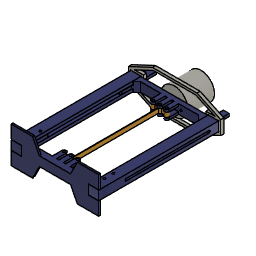
Modelo Pandeo De Columna (Autodesk Fusion 360 design; units mm, degrees)
Autodesk Fusion 360 part; units mm, degrees
note: some values were not read from the file. Set by a fixed rule: which sketch regions a step uses.
(part 1 of 2)
sketch "Boceto1" plane through (0, 0, 0) normal (0, 0, 1) x (1, 0, 0)
  circle A0 centre (0, 0) radius 2.65
  circle A1 centre (-15, 0) radius 2.65
  circle A2 centre (15, 0) radius 2.65
  circle A3 centre (0, 200) radius 2.65
  circle A4 centre (-15, 200) radius 2.65
  circle A5 centre (15, 200) radius 2.65
  line L0 (-15, 0) -> (15, 0) construction
  line L1 (-15, 200) -> (15, 200) construction
  line L2 (0, 0) -> (0, 200) construction
  line L3 (-0.5, 197.3976) -> (-0.5, 2.6024)
  line L4 (0.5, 2.6024) -> (0.5, 197.3976)
  line L5 (-12.5459, 201) -> (-2.4541, 201)
  line L6 (-12.5459, 199) -> (-2.4541, 199)
  line L7 (2.4541, 201) -> (12.5459, 201)
  line L8 (2.4541, 199) -> (12.5459, 199)
  line L9 (-12.5459, 1) -> (-2.4541, 1)
  line L10 (-12.5459, -1) -> (-2.4541, -1)
  line L11 (2.4541, 1) -> (12.5459, 1)
  line L12 (2.4541, -1) -> (12.5459, -1)
  circle A6 centre (-15, 200) radius 4.25
  circle A7 centre (0, 200) radius 4.25
  circle A8 centre (15, 200) radius 4.25
  circle A9 centre (-15, 0) radius 4.25
  circle A10 centre (0, 0) radius 4.25
  circle A11 centre (15, 0) radius 4.25
  dimension "d1" = 5.3
  dimension "d2" = 30
  dimension "d3" = 200
  dimension "Altura_Columna" = 200
  dimension "Ancho_Estructura" = 10
  dimension "Espesor_Columna" = 1
  dimension "d7" = 2
  dimension "d8" = 2
  dimension "d9" = 2
  dimension "d10" = 2
  dimension "d11" = 1
  dimension "d12" = 1.6
  dimension "d13" = 1.6
  dimension "d14" = 1.6
  dimension "d15" = 1.6
  dimension "d16" = 1.6
  dimension "d17" = 1.6
  dimension "Ancho_Columna" = 9.99
  constraint coincident A0.centre L2.start
  constraint equal A0 A1
  constraint equal A0 A2
  constraint equal A0 A3
  constraint equal A3 A4
  constraint equal A3 A5
  constraint coincident A1.centre L0.start
  constraint coincident A2.centre L0.end
  constraint coincident A4.centre L1.start
  constraint coincident A5.centre L1.end
  constraint horizontal L1
  constraint horizontal L0
  constraint coincident A0.centre L0
  constraint coincident A3.centre L1
  constraint equal L0 L1
  constraint coincident A3.centre L2.end
  constraint vertical L2
  constraint symmetric A1 A2 L2
  constraint symmetric A4 A5 L2
  constraint coincident A3 L3.start
  constraint coincident A0 L3.end
  constraint parallel L2 L3
  constraint coincident A0 L4.start
  constraint coincident A3 L4.end
  constraint parallel L2 L4
  constraint coincident A4 L5.start
  constraint coincident A3 L5.end
  constraint perpendicular L4 L5
  constraint coincident A4 L6.start
  constraint coincident A3 L6.end
  constraint parallel L5 L6
  constraint coincident A3 L7.start
  constraint coincident A5 L7.end
  constraint perpendicular L2 L7
  constraint coincident A3 L8.start
  constraint coincident A5 L8.end
  constraint perpendicular L2 L8
  constraint equal L5 L6
  constraint equal L7 L8
  constraint equal L3 L4
  constraint coincident A1 L9.start
  constraint coincident A0 L9.end
  constraint parallel L0 L9
  constraint coincident A1 L10.start
  constraint coincident A0 L10.end
  constraint parallel L0 L10
  constraint coincident A0 L11.start
  constraint coincident A2 L11.end
  constraint parallel L10 L11
  constraint coincident A0 L12.start
  constraint coincident A2 L12.end
  constraint parallel L0 L12
  constraint equal L9 L10
  constraint equal L11 L12
  measures "d1" diameter of A0
  measures "d2" distance of A1.centre A2.centre
  measures "d3" distance of A0.centre A3.centre
  measures "d7" distance of L5 L6
  measures "d8" distance of L7 L8
  measures "d9" distance of L11 L12
  measures "d10" distance of L9 L10
  measures "d11" distance of L3 L4
extrude "Extruir1" add sketch "Boceto1" along normal blind 10 contours A0 L11 L12 A10 | A0 L4 L11 A10 | A0 L10 L12 A10 | A0 L3 L4 A10 | L11 L12 A10 A11 | A0 L9 L10 A10 | A0 L3 L9 A10 | L3 L4 A7 A10 | A2 L11 L12 A11 | A2 L11 L12 A11 | L9 L10 A9 A10 | A3 L3 L4 A7 | A3 L4 L8 A7 | A1 L9 L10 A9 | A1 L9 L10 A9 | A3 L3 L6 A7 | L7 L8 A7 A8 | A3 L7 L8 A7 | A3 L5 L6 A7 | L5 L6 A6 A7 | A5 L7 L8 A8 | A5 L7 L8 A8 | A4 L5 L6 A6 | A4 L5 L6 A6 | A3 L5 L7 A7 makes body 1
ref_plane "PlanoDeObra1" through (0, 100, 10.4) normal (0, 0, 1) x (1, 0, 0)
sketch "Boceto2" plane through (0, 0, 10.4) normal (0, 0, 1) x (1, 0, 0)
  line L0 (10.8693, 1) -> (4.1307, 1)
  arc A0 (4.1307, 1) -> (0.5, 4.2205) centre (0, 0) ccw
  line L1 (0.5, 4.2205) -> (0.5, 195.7795)
  line L2 (-95, 221.5) -> (95, 221.5)
  line L3 (0, 200) -> (0, 221.5) construction
  line L4 (-95, -21.5) -> (95, -21.5)
  line L5 (0, 0) -> (0, -21.5) construction
  line L6 (-95, 221.5) -> (-95, 231.5)
  line L7 (-95, 231.5) -> (95, 231.5)
  line L8 (95, 231.5) -> (95, 221.5)
  line L9 (-95, -21.5) -> (-95, -31.5)
  line L10 (-95, -31.5) -> (95, -31.5)
  line L11 (95, -31.5) -> (95, -21.5)
  circle A1 centre (-15, 200) radius 5
  circle A2 centre (15, 200) radius 5
  circle A3 centre (0, 200) radius 5
  circle A4 centre (-15, 0) radius 5
  circle A5 centre (0, 0) radius 5
  circle A6 centre (15, 0) radius 5
  line L12 (-20, 0) -> (-10, 0) construction
  line L13 (-10, 0) -> (-10, -21.5)
  line L14 (-10, -21.5) -> (-20, -21.5)
  line L15 (-20, -21.5) -> (-20, 0)
  line L16 (-5, 0) -> (5, 0) construction
  line L17 (5, 0) -> (5, -21.5)
  line L18 (5, -21.5) -> (-5, -21.5)
  line L19 (-5, -21.5) -> (-5, 0)
  line L20 (10, 0) -> (20, 0) construction
  line L21 (20, 0) -> (20, -21.5)
  line L22 (20, -21.5) -> (10, -21.5)
  line L23 (10, -21.5) -> (10, 0)
  line L24 (-20, 200) -> (-10, 200) construction
  line L25 (-10, 200) -> (-10, 221.5)
  line L26 (-10, 221.5) -> (-20, 221.5)
  line L27 (-20, 221.5) -> (-20, 200)
  line L28 (-5, 200) -> (5, 200) construction
  line L29 (5, 200) -> (5, 221.5)
  line L30 (5, 221.5) -> (-5, 221.5)
  line L31 (-5, 221.5) -> (-5, 200)
  line L32 (10, 200) -> (20, 200) construction
  line L33 (20, 200) -> (20, 221.5)
  line L34 (20, 221.5) -> (10, 221.5)
  line L35 (10, 221.5) -> (10, 200)
  circle A7 centre (15, 200) radius 2.65
  circle A8 centre (-15, 200) radius 2.65
  circle A9 centre (0, 200) radius 2.65
  circle A10 centre (15, 0) radius 2.65
  circle A11 centre (-15, 0) radius 2.65
  circle A12 centre (0, 0) radius 2.65
  arc A13 (-10.8693, 1) -> (-10.8693, -1) centre (-15, 0) ccw
  line L36 (-10.8693, -1) -> (-4.1307, -1)
  arc A14 (-4.1307, -1) -> (4.1307, -1) centre (0, 0) ccw
  line L37 (4.1307, -1) -> (10.8693, -1)
  arc A15 (10.8693, -1) -> (10.8693, 1) centre (15, 0) ccw
  arc A16 (0.5, 195.7795) -> (4.1307, 199) centre (0, 200) ccw
  line L38 (4.1307, 199) -> (10.8693, 199)
  arc A17 (10.8693, 199) -> (10.8693, 201) centre (15, 200) ccw
  line L39 (10.8693, 201) -> (4.1307, 201)
  arc A18 (4.1307, 201) -> (-4.1307, 201) centre (0, 200) ccw
  line L40 (-4.1307, 201) -> (-10.8693, 201)
  arc A19 (-10.8693, 201) -> (-10.8693, 199) centre (-15, 200) ccw
  line L41 (-10.8693, 199) -> (-4.1307, 199)
  arc A20 (-4.1307, 199) -> (-0.5, 195.7795) centre (0, 200) ccw
  line L42 (-0.5, 195.7795) -> (-0.5, 4.2205)
  arc A21 (-0.5, 4.2205) -> (-4.1307, 1) centre (0, 0) ccw
  line L43 (-4.1307, 1) -> (-10.8693, 1)
  dimension "d21" = 21.5
  dimension "d22" = 190
  dimension "d23" = 21.5
  dimension "d24" = 10
  dimension "d25" = 10
  dimension "d26" = 10
  dimension "d27" = 10
  dimension "d28" = 10
  dimension "d29" = 10
  dimension "d30" = 10
  dimension "d31" = 10
  constraint horizontal L2
  constraint midpoint L2 L3.end
  constraint vertical L3
  constraint coincident A0.centre L5.start
  constraint midpoint L4 L5.end
  constraint vertical L5
  constraint equal L2 L4
  constraint perpendicular L2 L6
  constraint perpendicular L6 L7
  constraint perpendicular L2 L8
  constraint perpendicular L9 L10
  constraint perpendicular L4 L11
  constraint parallel L4 L10
  constraint horizontal L4
  constraint coincident L3.start A3.centre
  constraint horizontal L12
  constraint vertical L13
  constraint horizontal L14
  constraint vertical L15
  constraint coincident L4 L13.end
  constraint coincident A4 L12.start
  constraint horizontal L16
  constraint vertical L17
  constraint horizontal L18
  constraint vertical L19
  constraint coincident L4 L17.end
  constraint coincident A5 L16.start
  constraint horizontal L20
  constraint vertical L21
  constraint horizontal L22
  constraint vertical L23
  constraint coincident L4 L21.end
  constraint coincident A6 L20.start
  constraint coincident A4 L12.end
  constraint coincident A5 L16.end
  constraint coincident A6 L20.end
  constraint coincident A6.centre L20
  constraint coincident A0.centre L16
  constraint coincident A4.centre L12
  constraint horizontal L24
  constraint vertical L25
  constraint horizontal L26
  constraint vertical L27
  constraint coincident L2 L25.end
  constraint coincident A1 L24.start
  constraint horizontal L28
  constraint vertical L29
  constraint horizontal L30
  constraint vertical L31
  constraint coincident L2 L29.end
  constraint coincident A3 L28.start
  constraint horizontal L32
  constraint vertical L33
  constraint horizontal L34
  constraint vertical L35
  constraint coincident L2 L33.end
  constraint coincident A2 L32.start
  constraint coincident A2 L32.end
  constraint coincident A2.centre L32
  constraint coincident A3 L28.end
  constraint coincident L3.start L28
  constraint coincident A1.centre L24
  constraint coincident A1 L24.end
  constraint coincident A2.centre A7.centre
  constraint coincident A1.centre A8.centre
  constraint coincident A4.centre A11.centre
  constraint coincident A6.centre A10.centre
  measures "d21" distance of L2 L3.start
  measures "d22" distance of L2.start L2.end
  measures "d23" distance of A0.centre L5.end
  measures "d24" distance of L4 L10
  measures "d25" distance of L2 L7
  measures "d26" diameter of A1
  measures "d27" diameter of A2
  measures "d28" diameter of A3
  measures "d29" diameter of A4
  measures "d30" diameter of A5
  measures "d31" diameter of A6
extrude "Extruir2" add sketch "Boceto2" along normal blind 5 and the other way blind 15.8 separate body contours L4 L9 L10 L11 L14 L18 L22 | L2 L6 L7 L8 L26 L30 L34 makes body 2 at (-31.6667, -21.5, 1.5333) makes body 3 at (31.6667, 221.5, 8.4667)
sketch "Boceto7" plane through (0, 231.5, 0) normal (0, 1, 0) x (-1, 0, 0)
  line L0 (95, -5.4) -> (95, 15.4)
  line L1 (95, 15.4) -> (-95, 15.4)
  line L2 (-95, 15.4) -> (-95, -5.4)
  line L3 (-95, -5.4) -> (95, -5.4)
  line L4 (-95, -5.4) -> (95, 15.4) construction
  line L5 (-25, 5) -> (25, 5) construction
  circle A0 centre (-25, 5) radius 2.25
  circle A1 centre (25, 5) radius 2.25
  circle A2 centre (0, 5) radius 30
  point P0 (0, 5)
  dimension "d63" = 50
  dimension "d64" = 4.5
  dimension "d65" = 4.5
  dimension "d68" = 60
  constraint coincident L2.end L3.start
  constraint coincident L0.end L1.start
  constraint midpoint L5 P0
  constraint midpoint L4 P0
  constraint horizontal L5
  constraint coincident L5.start A0.centre
  constraint coincident L5.end A1.centre
  constraint coincident P0 A2.centre
  measures "d63" distance of L5.start L5.end
  measures "d64" diameter of A0
  measures "d65" diameter of A1
  measures "d68" diameter of A2
extrude "Extruir11" add sketch "Boceto7" along normal blind 60 separate body contours L3 A2 | L1 L3 A2 | L1 A2 | A0 | A1 makes body 4
shell "Vaciado1" thickness 1.6 removed faces 1 at (9.9749, 291.5, 4.2926) on bodies 4
extrude "Extruir12" cut sketch "Boceto7" along normal blind 7 contours A0 | A1 bodies 4
extrude "Extruir3" add sketch "Boceto2" against normal up to surface (5 mm away) from surface at -10.8 contours L0 A6 L37 A15 | L0 A6 L37 A15 | L0 A0 L1 A5 L36 A14 L37 L42 A21 L43 | L0 A0 L1 A5 | L4 A6 L21 L22 L23 L37 | A6 L23 L37 | A5 L17 L37 | L4 A5 L17 L18 L19 L36 L37 | A5 L36 A14 L37 | L1 A3 A16 L38 L39 A18 L40 L41 A20 L42 | L1 A3 A16 L38 | A5 L42 A21 L43 | A5 L19 L36 | A3 L41 A20 L42 | A3 L29 L39 | A2 L38 A17 L39 | A2 L38 A17 L39 | A4 A13 L36 L43 | A4 A13 L36 L43 | A4 L13 L36 | L4 A4 L13 L14 L15 L36 | A3 L31 L40 | A1 L40 A19 L41 | A1 L40 A19 L41 | A3 L39 A18 L40 | L2 A3 L29 L30 L31 L39 L40 | A2 L35 L39 | L2 A2 L33 L34 L35 L39 | L2 A1 L25 L26 L27 L40 | A1 L25 L40 bodies 2 3
extrude "Extruir4" add sketch "Boceto2" along normal up to surface (5 mm away) contours L0 A6 L37 A15 | L0 A6 L37 A15 | L0 A0 L1 A5 L36 A14 L37 L42 A21 L43 | L0 A0 L1 A5 | L4 A6 L21 L22 L23 L37 | A6 L23 L37 | A5 L17 L37 | L4 A5 L17 L18 L19 L36 L37 | A5 L36 A14 L37 | L1 A3 A16 L38 L39 A18 L40 L41 A20 L42 | L1 A3 A16 L38 | A5 L42 A21 L43 | A5 L19 L36 | A3 L41 A20 L42 | A3 L29 L39 | A2 L38 A17 L39 | A2 L38 A17 L39 | A4 A13 L36 L43 | A4 A13 L36 L43 | A4 L13 L36 | L4 A4 L13 L14 L15 L36 | A3 L31 L40 | A1 L40 A19 L41 | A1 L40 A19 L41 | A3 L39 A18 L40 | L2 A3 L29 L30 L31 L39 L40 | A2 L35 L39 | L2 A2 L33 L34 L35 L39 | L2 A1 L25 L26 L27 L40 | A1 L25 L40 bodies 2 3
sketch "Boceto17" plane through (0, -31.5, 0) normal (0, -1, 0) x (1, 0, 0)
  line L0 (95, -5.4) -> (95, 15.4)
  line L1 (95, 15.4) -> (-95, 15.4)
  line L2 (-95, 15.4) -> (-95, -5.4)
  line L3 (-95, -5.4) -> (95, -5.4)
  line L4 (-75, 15.4) -> (-95, 15.4)
  line L5 (-95, 15.4) -> (-95, 8.4667)
  line L6 (-95, 8.4667) -> (-75, 8.4667)
  line L7 (-75, 8.4667) -> (-75, 15.4)
  line L8 (-75, -5.4) -> (-95, -5.4)
  line L9 (-95, -5.4) -> (-95, 1.5333)
  line L10 (-95, 1.5333) -> (-75, 1.5333)
  line L11 (-75, 1.5333) -> (-75, -5.4)
  line L12 (-88.0667, 8.4667) -> (-95, 8.4667)
  line L13 (-95, 8.4667) -> (-95, 1.5333)
  line L14 (-95, 1.5333) -> (-88.0667, 1.5333)
  line L15 (-88.0667, 1.5333) -> (-88.0667, 8.4667)
  line L16 (-88.0667, 1.5333) -> (-95, 8.4667)
  line L17 (95, 15.4) -> (75, 15.4)
  line L18 (75, 15.4) -> (75, 8.4667)
  line L19 (75, 8.4667) -> (95, 8.4667)
  line L20 (95, 8.4667) -> (95, 15.4)
  line L21 (95, -5.4) -> (75, -5.4)
  line L22 (75, -5.4) -> (75, 1.5333)
  line L23 (75, 1.5333) -> (95, 1.5333)
  line L24 (95, 1.5333) -> (95, -5.4)
  line L25 (88.0667, 1.5333) -> (95, 1.5333)
  line L26 (95, 1.5333) -> (95, 8.4667)
  line L27 (95, 8.4667) -> (88.0667, 8.4667)
  line L28 (88.0667, 8.4667) -> (88.0667, 1.5333)
  line L29 (88.0667, 1.5333) -> (95, 8.4667)
  dimension "d100" = 45
  dimension "d101" = 45
  dimension "d119" = 20
  dimension "d120" = 20
  constraint horizontal L4
  constraint vertical L5
  constraint horizontal L6
  constraint vertical L7
  constraint coincident L2 L5.end
  constraint coincident L1 L4.start
  constraint horizontal L8
  constraint vertical L9
  constraint horizontal L10
  constraint vertical L11
  constraint coincident L2 L9.end
  constraint coincident L3 L8.start
  constraint horizontal L12
  constraint vertical L13
  constraint horizontal L14
  constraint vertical L15
  constraint equal L7 L15
  constraint equal L11 L15
  constraint equal L6 L10
  constraint horizontal L17
  constraint vertical L18
  constraint horizontal L19
  constraint vertical L20
  constraint coincident L0.end L1.start
  constraint horizontal L21
  constraint vertical L22
  constraint horizontal L23
  constraint vertical L24
  constraint coincident L0.start L3.end
  constraint horizontal L25
  constraint vertical L26
  constraint horizontal L27
  constraint vertical L28
  constraint equal L18 L22
  constraint equal L18 L28
  constraint equal L19 L23
  constraint coincident L6 L12.start
  constraint coincident L23 L25.start
  measures "d100" angle of L10 L16
  measures "d101" angle of L23 L29
  measures "d119" distance of L5.end L6.end
  measures "d120" distance of L18.end L19.end
extrude "Extruir24" cut sketch "Boceto17" against normal blind 285 contours L0 L3 L21 L22 L23 L24 L25 | L0 L23 L25 L26 L29 | L0 L1 L17 L18 L19 L20 L27 | L19 L27 L28 L29 | L2 L3 L8 L9 L10 L11 L14 | L2 L10 L13 L14 L16 | L6 L12 L15 L16 | L1 L2 L4 L5 L6 L7 L12 bodies 2 3
sketch "Boceto18" plane through (0, 221.5, 0) normal (0, -1, 0) x (1, 0, 0)
  line L0 (-75, 15.4) -> (-75, 8.4667)
  line L1 (-75, 8.4667) -> (-88.0667, 8.4667)
  line L2 (-88.0667, 8.4667) -> (-88.0667, 1.5333)
  line L3 (-88.0667, 1.5333) -> (-75, 1.5333)
  line L4 (-75, 1.5333) -> (-75, -5.4)
  line L5 (-75, -5.4) -> (-20, -5.4)
  line L6 (-20, -5.4) -> (-20, -0.4)
  line L7 (-20, -0.4) -> (-10, -0.4)
  line L8 (-10, -0.4) -> (-10, -5.4)
  line L9 (-10, -5.4) -> (-5, -5.4)
  line L10 (-5, -5.4) -> (-5, -0.4)
  line L11 (-5, -0.4) -> (5, -0.4)
  line L12 (5, -0.4) -> (5, -5.4)
  line L13 (5, -5.4) -> (10, -5.4)
  line L14 (10, -5.4) -> (10, -0.4)
  line L15 (10, -0.4) -> (20, -0.4)
  line L16 (20, -0.4) -> (20, -5.4)
  line L17 (20, -5.4) -> (75, -5.4)
  line L18 (75, -5.4) -> (75, 1.5333)
  line L19 (75, 1.5333) -> (88.0667, 1.5333)
  line L20 (88.0667, 1.5333) -> (88.0667, 8.4667)
  line L21 (88.0667, 8.4667) -> (75, 8.4667)
  line L22 (75, 8.4667) -> (75, 15.4)
  line L23 (75, 15.4) -> (20, 15.4)
  line L24 (20, 15.4) -> (20, 10.4)
  line L25 (20, 10.4) -> (10, 10.4)
  line L26 (10, 10.4) -> (10, 15.4)
  line L27 (10, 15.4) -> (5, 15.4)
  line L28 (5, 15.4) -> (5, 10.4)
  line L29 (5, 10.4) -> (-5, 10.4)
  line L30 (-5, 10.4) -> (-5, 15.4)
  line L31 (-5, 15.4) -> (-10, 15.4)
  line L32 (-10, 15.4) -> (-10, 10.4)
  line L33 (-10, 10.4) -> (-20, 10.4)
  line L34 (-20, 10.4) -> (-20, 15.4)
  line L35 (-20, 15.4) -> (-75, 15.4)
  line L36 (-88.0667, 8.4667) -> (-75, 8.4667)
  line L37 (-75, 8.4667) -> (-75, 1.5333)
  line L38 (-75, 1.5333) -> (-88.0667, 1.5333)
  line L39 (-88.0667, 1.5333) -> (-88.0667, 8.4667)
  line L40 (88.0667, 8.4667) -> (75, 8.4667)
  line L41 (75, 8.4667) -> (75, 1.5333)
  line L42 (75, 1.5333) -> (88.0667, 1.5333)
  line L43 (88.0667, 1.5333) -> (88.0667, 8.4667)
  constraint horizontal L36
  constraint vertical L37
  constraint horizontal L38
  constraint vertical L39
  constraint coincident L3.end L4.start
  constraint coincident L1.end L2.start
  constraint horizontal L40
  constraint vertical L41
  constraint horizontal L42
  constraint vertical L43
  constraint coincident L18.end L19.start
  constraint coincident L20.end L21.start
extrude "Extruir25" add sketch "Boceto18" along normal blind 35 contours L1 L2 L3 L36 L37 L38 L39 | L19 L20 L21 L40 L41 L42 L43 bodies 3
chamfer "Chaflán1" distance 10 angle 45 2 edges at (-75, 221.5, 5) (75, 221.5, 5) on bodies 3
sketch "Boceto19" plane through (0, -31.5, 0) normal (0, -1, 0) x (1, 0, 0)
  line L0 (-75, 1.5333) -> (-75, -5.4)
  line L1 (-75, -5.4) -> (75, -5.4)
  line L2 (75, -5.4) -> (75, 1.5333)
  line L3 (75, 1.5333) -> (88.0667, 1.5333)
  line L4 (88.0667, 1.5333) -> (88.0667, 8.4667)
  line L5 (88.0667, 8.4667) -> (75, 8.4667)
  line L6 (75, 8.4667) -> (75, 15.4)
  line L7 (75, 15.4) -> (-75, 15.4)
  line L8 (-75, 15.4) -> (-75, 8.4667)
  line L9 (-75, 8.4667) -> (-88.0667, 8.4667)
  line L10 (-88.0667, 8.4667) -> (-88.0667, 1.5333)
  line L11 (-88.0667, 1.5333) -> (-75, 1.5333)
  line L12 (-75.15, 8.6167) -> (-88.2167, 8.6167)
  line L13 (-88.2167, 8.6167) -> (-88.2167, 1.3833)
  line L14 (-88.2167, 1.3833) -> (-75.15, 1.3833)
  line L15 (-75.15, 1.3833) -> (-75.15, -5.55)
  line L16 (-75.15, -5.55) -> (75.15, -5.55)
  line L17 (75.15, -5.55) -> (75.15, 1.3833)
  line L18 (75.15, 1.3833) -> (88.2167, 1.3833)
  line L19 (88.2167, 1.3833) -> (88.2167, 8.6167)
  line L20 (88.2167, 8.6167) -> (75.15, 8.6167)
  line L21 (75.15, 8.6167) -> (75.15, 15.55)
  line L22 (75.15, 15.55) -> (-75.15, 15.55)
  line L23 (-75.15, 15.55) -> (-75.15, 8.6167)
  line L24 (75, 15.4) -> (98.0667, 15.4)
  line L25 (98.0667, 15.4) -> (98.0667, -5.4)
  line L26 (98.0667, -5.4) -> (75, -5.4)
  dimension "d107" = 0.15
  dimension "d108" = 10
  constraint coincident L6.end L7.start
  constraint perpendicular L21 L24
  constraint perpendicular L24 L25
  constraint coincident L1.end L2.start
  constraint parallel L24 L26
  measures "d108" distance of L4 L25
extrude "Extruir26" add sketch "Boceto19" against normal blind 270 separate body contours L17 L18 L19 L20 L21 L24 L25 L26 makes body 5
sketch "Boceto20" plane through (0, 0, 8.4667) normal (0, 0, 1) x (-1, 0, 0)
  line L0 (-88.0667, 21.5) -> (-75, 21.5)
  line L1 (-75, 21.5) -> (-75, 31.5)
  line L2 (-75, 31.5) -> (-88.0667, 31.5)
  line L3 (-88.0667, 31.5) -> (-88.0667, 21.5)
  line L4 (-75, 21.5) -> (-88.0667, 21.5)
  line L5 (-88.0667, 21.5) -> (-88.0667, 31.5)
  line L6 (-88.0667, 31.5) -> (-75, 31.5)
  line L7 (-75, 31.5) -> (-75, 21.5)
  line L8 (-88.0667, 31.5) -> (-75, 21.5)
  circle A0 centre (-81.5333, 26.5) radius 2.65
  circle A1 centre (-81.5333, 6.5) radius 2.65
  dimension "d111" = 5.3
  dimension "d133" = 0
  dimension "d134" = -20
  constraint coincident L2.end L3.start
  constraint coincident L0.end L1.start
  constraint midpoint L8 A0.centre
  measures "d111" diameter of A0
extrude "Extruir27" cut sketch "Boceto20" along normal blind 8 and the other way blind 22 contours L8 A0 | L8 A0 bodies 2 5
sketch "Boceto21" plane through (0, -21.5, 0) normal (0, 1, 0) x (-1, 0, 0)
  line L0 (75, -5.4) -> (75, 1.5333)
  line L1 (75, 1.5333) -> (88.0667, 1.5333)
  line L2 (88.0667, 1.5333) -> (88.0667, 8.4667)
  line L3 (88.0667, 8.4667) -> (75, 8.4667)
  line L4 (75, 8.4667) -> (75, 15.4)
  line L5 (75, 15.4) -> (20, 15.4)
  line L6 (20, 15.4) -> (20, 10.4)
  line L7 (20, 10.4) -> (10, 10.4)
  line L8 (10, 10.4) -> (10, 15.4)
  line L9 (10, 15.4) -> (5, 15.4)
  line L10 (5, 15.4) -> (5, 10.4)
  line L11 (5, 10.4) -> (-5, 10.4)
  line L12 (-5, 10.4) -> (-5, 15.4)
  line L13 (-5, 15.4) -> (-10, 15.4)
  line L14 (-10, 15.4) -> (-10, 10.4)
  line L15 (-10, 10.4) -> (-20, 10.4)
  line L16 (-20, 10.4) -> (-20, 15.4)
  line L17 (-20, 15.4) -> (-75, 15.4)
  line L18 (-75, 15.4) -> (-75, 8.4667)
  line L19 (-75, 8.4667) -> (-88.0667, 8.4667)
  line L20 (-88.0667, 8.4667) -> (-88.0667, 1.5333)
  line L21 (-88.0667, 1.5333) -> (-75, 1.5333)
  line L22 (-75, 1.5333) -> (-75, -5.4)
  line L23 (-75, -5.4) -> (-20, -5.4)
  line L24 (-20, -5.4) -> (-20, -0.4)
  line L25 (-20, -0.4) -> (-10, -0.4)
  line L26 (-10, -0.4) -> (-10, -5.4)
  line L27 (-10, -5.4) -> (-5, -5.4)
  line L28 (-5, -5.4) -> (-5, -0.4)
  line L29 (-5, -0.4) -> (5, -0.4)
  line L30 (5, -0.4) -> (5, -5.4)
  line L31 (5, -5.4) -> (10, -5.4)
  line L32 (10, -5.4) -> (10, -0.4)
  line L33 (10, -0.4) -> (20, -0.4)
  line L34 (20, -0.4) -> (20, -5.4)
  line L35 (20, -5.4) -> (75, -5.4)
  line L36 (-88.0667, 1.5333) -> (-75, 1.5333)
  line L37 (-75, 1.5333) -> (-75, 8.4667)
  line L38 (-75, 8.4667) -> (-88.0667, 8.4667)
  line L39 (-88.0667, 8.4667) -> (-88.0667, 1.5333)
  line L40 (75, 1.5333) -> (88.0667, 1.5333)
  line L41 (88.0667, 1.5333) -> (88.0667, 8.4667)
  line L42 (88.0667, 8.4667) -> (75, 8.4667)
  line L43 (75, 8.4667) -> (75, 1.5333)
  constraint horizontal L36
  constraint vertical L37
  constraint horizontal L38
  constraint vertical L39
  constraint coincident L18.end L19.start
  constraint coincident L20.end L21.start
  constraint horizontal L40
  constraint vertical L41
  constraint horizontal L42
  constraint vertical L43
  constraint coincident L2.end L3.start
  constraint coincident L0.end L1.start
extrude "Extruir28" add sketch "Boceto21" along normal blind 45 contours L1 L2 L3 L40 L41 L42 L43 | L19 L20 L21 L36 L37 L38 L39 bodies 2
chamfer "Chaflán2" distance 10 angle 45 2 edges at (75, -21.5, 5) (-75, -21.5, 5) on bodies 2
mirror "Simetría1" about plane through (0, 0, 0) normal (1, 0, 0) of bodies 5 makes body 6
mirror "Simetría2" about plane through (0, 0, 0) normal (1, 0, 0) of "Extruir27"
sketch "Boceto22" plane through (0, -31.5, 0) normal (0, -1, 0) x (1, 0, 0)
  line L0 (-75, 1.5333) -> (-75, -5.4)
  line L1 (-75, -5.4) -> (75, -5.4)
  line L2 (75, -5.4) -> (75, 1.5333)
  line L3 (75, 1.5333) -> (88.0667, 1.5333)
  line L4 (88.0667, 1.5333) -> (88.0667, 8.4667)
  line L5 (88.0667, 8.4667) -> (75, 8.4667)
  line L6 (75, 8.4667) -> (75, 15.4)
  line L7 (75, 15.4) -> (-75, 15.4)
  line L8 (-75, 15.4) -> (-75, 8.4667)
  line L9 (-75, 8.4667) -> (-88.0667, 8.4667)
  line L10 (-88.0667, 8.4667) -> (-88.0667, 1.5333)
  line L11 (-88.0667, 1.5333) -> (-75, 1.5333)
  line L12 (-75, 15.4) -> (75, 15.4)
  line L13 (75, 15.4) -> (75, -5.4)
  line L14 (75, -5.4) -> (-75, -5.4)
  line L15 (-75, -5.4) -> (-75, 15.4)
  constraint horizontal L12
  constraint vertical L13
  constraint horizontal L14
  constraint vertical L15
  constraint coincident L1.end L2.start
  constraint coincident L7.end L8.start
extrude "Extruir29" add sketch "Boceto22" along normal blind 4 contours L0 L1 L2 L6 L7 L8 L12 L13 L14 L15 bodies 2
extrude "Extruir30" add 2 faces at (94.7833, -31.5, 3.7944) (-94.7833, -31.5, 3.7944) along direction (0, -1, 0) blind 0.2 on bodies 5 6 bodies 5 6
sketch "Boceto23" plane through (0, -31.7, 0) normal (0, -1, 0) x (1, 0, 0)
  line L0 (-98.0667, 15.4) -> (-98.0667, -5.4)
  line L1 (-98.0667, -5.4) -> (-75.15, -5.4)
  line L2 (-75.15, -5.4) -> (-75.15, 1.3833)
  line L3 (-75.15, 1.3833) -> (-88.2167, 1.3833)
  line L4 (-88.2167, 1.3833) -> (-88.2167, 8.6167)
  line L5 (-88.2167, 8.6167) -> (-75.15, 8.6167)
  line L6 (-75.15, 8.6167) -> (-75.15, 15.4)
  line L7 (-75.15, 15.4) -> (-98.0667, 15.4)
  line L8 (98.0667, -5.4) -> (98.0667, 15.4)
  line L9 (98.0667, 15.4) -> (75.15, 15.4)
  line L10 (75.15, 15.4) -> (75.15, 8.6167)
  line L11 (75.15, 8.6167) -> (88.2167, 8.6167)
  line L12 (88.2167, 8.6167) -> (88.2167, 1.3833)
  line L13 (88.2167, 1.3833) -> (75.15, 1.3833)
  line L14 (75.15, 1.3833) -> (75.15, -5.4)
  line L15 (75.15, -5.4) -> (98.0667, -5.4)
  line L16 (75.15, 8.6167) -> (75.15, 1.3833)
  line L17 (-75.15, 8.6167) -> (-75.15, 1.3833)
  constraint coincident L10.end L11.start
  constraint coincident L13.end L14.start
  constraint coincident L5.end L6.start
  constraint coincident L2.end L3.start
extrude "Extruir31" add sketch "Boceto23" along normal up to surface (3.8 mm away) bodies 5 6
sketch "Boceto24" plane through (0, 0, 15.4) normal (0, 0, 1) x (-1, 0, 0)
  circle A0 centre (-81.5333, 26.5) radius 2.65
  line L0 (-98.0667, 35.5) -> (-98.0667, -238.5)
  line L1 (-98.0667, -238.5) -> (-75.15, -238.5)
  line L2 (-75.15, -238.5) -> (-75.15, 35.5)
  line L3 (-75.15, 35.5) -> (-98.0667, 35.5)
  circle A1 centre (-81.5333, 6.5) radius 2.65
  circle A2 centre (81.5333, 6.5) radius 2.65
  line L4 (-81.5333, 26.5) -> (-81.5333, 6.5)
  circle A3 centre (81.5333, 26.5) radius 2.65
  line L5 (81.5333, 26.5) -> (81.5333, 6.5)
  dimension "d135" = 5.3
  dimension "d136" = 5.3
  dimension "d137" = 20
  dimension "d138" = 20
  constraint coincident A0.centre L4.start
  constraint coincident A1.centre L4.end
  constraint coincident A3.centre L5.start
  constraint coincident A2.centre L5.end
  constraint vertical L5
  constraint vertical L4
  measures "d135" diameter of A2
  measures "d136" diameter of A1
  measures "d137" distance of A0.centre A1.centre
  measures "d138" distance of A3.centre A2.centre
extrude "Extruir32" cut sketch "Boceto24" against normal blind 35 contours A1 | A2 bodies 2 5 6
sketch "Boceto25" plane through (0, 231.5, 0) normal (0, 1, 0) x (-1, 0, 0)
  line L0 (75, 8.4667) -> (75, 15.4)
  line L1 (75, 15.4) -> (-75, 15.4)
  line L2 (-75, 15.4) -> (-75, 8.4667)
  line L3 (-75, 8.4667) -> (-88.0667, 8.4667)
  line L4 (-88.0667, 8.4667) -> (-88.0667, 1.5333)
  line L5 (-88.0667, 1.5333) -> (-75, 1.5333)
  line L6 (-75, 1.5333) -> (-75, -5.4)
  line L7 (-75, -5.4) -> (75, -5.4)
  line L8 (75, -5.4) -> (75, 1.5333)
  line L9 (75, 1.5333) -> (88.0667, 1.5333)
  line L10 (88.0667, 1.5333) -> (88.0667, 8.4667)
  line L11 (88.0667, 8.4667) -> (75, 8.4667)
sketch "Boceto26" plane through (0, 231.5, 0) normal (0, 1, 0) x (-1, 0, 0)
  line L0 (75, -5) -> (-75, 15)
  line L1 (-75, 15) -> (0, 5)
  circle A0 centre (0, 5) radius 2.15
  circle A1 centre (-25, 5) radius 2.15
  circle A2 centre (25, 5) radius 2.15
  dimension "d146" = 4.3
  dimension "d149" = 25
  dimension "d150" = 0
  constraint midpoint L0 L1.end
  constraint coincident L1.end A0.centre
  measures "d146" diameter of A0
extrude "Extruir33" cut sketch "Boceto26" against normal blind 10 contours A1 | A2 bodies 3
sketch "Boceto27" plane through (0.5, 0, 0) normal (1, 0, 0) x (0, 1, 0)
  line L0 (4.2205, 0) -> (195.7795, 0)
  line L1 (195.7795, 0) -> (195.7795, 10)
  line L2 (195.7795, 10) -> (4.2205, 10)
  line L3 (4.2205, 10) -> (4.2205, 0)
  line L4 (195.7795, 5) -> (4.2205, 5) construction
  line L5 (195.7795, 0.005) -> (4.2205, 0.005)
  line L6 (4.2205, 0.005) -> (4.2205, 9.995)
  line L7 (4.2205, 9.995) -> (195.7795, 9.995)
  line L8 (195.7795, 9.995) -> (195.7795, 0.005)
  line L9 (195.7795, 0.005) -> (4.2205, 9.995) construction
  line L10 (4.2205, 0.005) -> (195.7795, 9.995) construction
  point P0 (100, 5)
  dimension "d153" = 9.99
  constraint midpoint L1 L4.start
  constraint midpoint L3 L4.end
  constraint horizontal L5
  constraint perpendicular L5 L6
  constraint parallel L5 L7
  constraint parallel L6 L8
  constraint coincident L9 P0
  constraint coincident L10 P0
  constraint coincident L1 L5.start
  constraint midpoint L4 P0
  measures "d153" distance of L5 L7
extrude "Extruir34" cut sketch "Boceto27" against normal blind 1 contours L0 L1 L3 L5 | L1 L2 L3 L7 bodies 1
sketch "Boceto28" plane through (0, 231.5, 0) normal (0, 1, 0) x (-1, 0, 0)
  line L0 (88.0667, 1.5333) -> (75, 1.5333)
  line L1 (75, 1.5333) -> (75, 8.4667)
  line L2 (75, 8.4667) -> (88.0667, 8.4667)
  line L3 (88.0667, 8.4667) -> (88.0667, 1.5333)
  line L4 (-88.0667, 1.5333) -> (-88.0667, 8.4667)
  line L5 (-88.0667, 8.4667) -> (-75, 8.4667)
  line L6 (-75, 8.4667) -> (-75, 1.5333)
  line L7 (-75, 1.5333) -> (-88.0667, 1.5333)
extrude "Extruir35" add sketch "Boceto28" along normal blind 35 bodies 3
chamfer "Chaflán3" distance 10 angle 45 2 edges at (-75, 231.5, 5) (75, 231.5, 5) on bodies 3
sketch "Boceto29" plane through (0, 0, 15.4) normal (0, 0, 1) x (-1, 0, 0)
  circle A0 centre (81.5333, 6.5) radius 2.65
  circle A1 centre (81.5333, 26.5) radius 2.65
  line L0 (75.15, 35.5) -> (75.15, -238.5)
  line L1 (75.15, -238.5) -> (98.0667, -238.5)
  line L2 (98.0667, -238.5) -> (98.0667, 35.5)
  line L3 (98.0667, 35.5) -> (75.15, 35.5)
  circle A2 centre (81.5333, -13.5) radius 2.65
  line L4 (81.5333, 6.5) -> (81.5333, -13.5)
  line L5 (81.5333, -13.5) -> (78.0407, -13.5)
  circle A3 centre (-81.5333, 6.5) radius 2.65
  circle A4 centre (-81.5333, 26.5) radius 2.65
  line L6 (-98.0667, 35.5) -> (-98.0667, -238.5)
  line L7 (-98.0667, -238.5) -> (-75.15, -238.5)
  line L8 (-75.15, -238.5) -> (-75.15, 35.5)
  line L9 (-75.15, 35.5) -> (-98.0667, 35.5)
  line L10 (-81.5333, 6.5) -> (-81.5333, -13.5)
  circle A5 centre (-81.5333, -13.5) radius 2.65
  dimension "d160" = 20
  dimension "d161" = 5.3
  dimension "d162" = 20
  dimension "d163" = 5.3
  constraint coincident A0.centre L4.start
  constraint coincident A2.centre L4.end
  constraint vertical L4
  constraint perpendicular L4 L5
  constraint coincident A3.centre L10.start
  constraint parallel L8 L10
  constraint coincident L10.end A5.centre
  measures "d160" distance of A0.centre A2.centre
  measures "d161" diameter of A2
  measures "d162" distance of A3.centre L10.end
  measures "d163" diameter of A5
extrude "Extruir36" cut sketch "Boceto29" against normal blind 30 contours A2 L4 L5 | A2 L4 L5 | A5 bodies 2 5 6
sketch "Boceto30" plane through (98.0667, 0, 0) normal (1, 0, 0) x (0, 1, 0)
  line L0 (-35.5, -5.4) -> (238.5, -5.4)
  line L1 (238.5, -5.4) -> (238.5, 15.4)
  line L2 (238.5, 15.4) -> (-35.5, 15.4)
  line L3 (-35.5, 15.4) -> (-35.5, -5.4)
  line L4 (-31.7, 8.6167) -> (238.5, 8.6167)
  line L5 (238.5, 8.6167) -> (238.5, 1.3833)
  line L6 (238.5, 1.3833) -> (-31.7, 1.3833)
  line L7 (-31.7, 1.3833) -> (-31.7, 8.6167)
  line L8 (211.5, 8.4667) -> (211.5, 1.5333)
  line L9 (211.5, 1.5333) -> (186.5, 1.5333)
  line L10 (186.5, 1.5333) -> (186.5, 8.4667)
  line L11 (186.5, 8.4667) -> (211.5, 8.4667)
  line L12 (-11.5, 1.5333) -> (-11.5, 8.4667)
  line L13 (-11.5, 8.4667) -> (23.5, 8.4667)
  line L14 (23.5, 8.4667) -> (23.5, 1.5333)
  line L15 (23.5, 1.5333) -> (-11.5, 1.5333)
  circle A0 centre (211.5, 5) radius 2.5
  circle A1 centre (26, 5) radius 2.5
  line L16 (23.5, 5) -> (211.5, 5)
  line L17 (26, 2.5) -> (211.5, 2.5)
  line L18 (211.5, 7.5) -> (26, 7.5)
  dimension "d166" = 5
  dimension "d167" = 5
  constraint midpoint L14 L16.start
  constraint midpoint L8 A0.centre
  constraint coincident A0.centre L16.end
  constraint coincident A1 L16.start
  constraint coincident A1.centre L16
  constraint coincident A1 L17.start
  constraint coincident A0 L17.end
  constraint perpendicular L8 L17
  constraint coincident A0 L18.start
  constraint coincident A1 L18.end
  constraint parallel L16 L18
  constraint tangent A1 L18
  constraint tangent A1 L17
  measures "d166" diameter of A0
  measures "d167" diameter of A1
extrude "Extruir37" cut sketch "Boceto30" against normal blind 280 contours L8 A0 | L8 A0 L16 | L10 A0 L16 L18 | L8 A0 L16 | L10 A0 L16 L17 | L10 A1 L16 L18 | L10 A1 L16 L17 | A1 L16 | A1 L16 bodies 5 6
sketch "Boceto31" plane through (88.0667, 0, 0) normal (1, 0, 0) x (0, 1, 0)
  line L0 (186.5, 1.5333) -> (266.5, 1.5333)
  line L1 (266.5, 1.5333) -> (266.5, 8.4667)
  line L2 (266.5, 8.4667) -> (186.5, 8.4667)
  line L3 (186.5, 8.4667) -> (186.5, 1.5333)
  arc A0 (211.5, 2.5) -> (211.5, 7.5) centre (211.5, 5) ccw
  line L4 (211.5, 2.5) -> (26, 2.5)
  line L5 (26, 7.5) -> (211.5, 7.5)
  line L6 (211.5, 5) -> (186.5, 5)
  circle A1 centre (199, 5) radius 2.15
  dimension "d170" = 4.3
  constraint coincident A0.centre L6.start
  constraint midpoint L3 L6.end
  constraint midpoint L6 A1.centre
  measures "d170" diameter of A1
extrude "Extruir38" [suppressed]
sketch "Boceto32" plane through (0, 0, 1.5333) normal (0, 0, -1) x (1, 0, 0)
  line L0 (75, -221.5) -> (75, -231.5)
  line L1 (75, -231.5) -> (65, -231.5)
  line L2 (65, -231.5) -> (75, -241.5)
  line L3 (75, -241.5) -> (75, -266.5)
  line L4 (75, -266.5) -> (88.0667, -266.5)
  line L5 (88.0667, -266.5) -> (88.0667, -186.5)
  line L6 (88.0667, -186.5) -> (75, -186.5)
  line L7 (75, -186.5) -> (75, -211.5)
  line L8 (75, -211.5) -> (65, -221.5)
  line L9 (65, -221.5) -> (75, -221.5)
  line L10 (-88.0667, -186.5) -> (-88.0667, -266.5)
  line L11 (-88.0667, -266.5) -> (-75, -266.5)
  line L12 (-75, -266.5) -> (-75, -241.5)
  line L13 (-75, -241.5) -> (-65, -231.5)
  line L14 (-65, -231.5) -> (-75, -231.5)
  line L15 (-75, -231.5) -> (-75, -221.5)
  line L16 (-75, -221.5) -> (-65, -221.5)
  line L17 (-65, -221.5) -> (-75, -211.5)
  line L18 (-75, -211.5) -> (-75, -186.5)
  line L19 (-75, -186.5) -> (-88.0667, -186.5)
  circle A0 centre (81.5333, -13.5) radius 2.65
  circle A1 centre (81.5333, 6.5) radius 2.65
  circle A2 centre (81.5333, 26.5) radius 2.65
  line L20 (88.0667, -23.5) -> (88.0667, 31.5)
  line L21 (88.0667, 31.5) -> (75, 31.5)
  line L22 (75, 31.5) -> (75, 21.5)
  line L23 (75, 21.5) -> (65, 21.5)
  line L24 (65, 21.5) -> (75, 11.5)
  line L25 (75, 11.5) -> (75, -23.5)
  line L26 (75, -23.5) -> (88.0667, -23.5)
  circle A3 centre (-81.5333, -13.5) radius 2.65
  circle A4 centre (-81.5333, 6.5) radius 2.65
  circle A5 centre (-81.5333, 26.5) radius 2.65
  line L27 (-75, 21.5) -> (-75, 31.5)
  line L28 (-75, 31.5) -> (-88.0667, 31.5)
  line L29 (-88.0667, 31.5) -> (-88.0667, -23.5)
  line L30 (-88.0667, -23.5) -> (-75, -23.5)
  line L31 (-75, -23.5) -> (-75, 11.5)
  line L32 (-75, 11.5) -> (-65, 21.5)
  line L33 (-65, 21.5) -> (-75, 21.5)
  line L34 (75, -241.5) -> (75, -211.5)
  line L35 (-75, -241.5) -> (-75, -211.5)
  line L36 (-75, 11.5) -> (-75, 21.5)
  line L37 (75, 11.5) -> (75, 21.5)
  constraint coincident L2.end L3.start
  constraint coincident L7.end L8.start
  constraint coincident L12.end L13.start
  constraint coincident L17.end L18.start
  constraint coincident L31.end L32.start
  constraint coincident L27.start L33.end
  constraint coincident L24.end L25.start
  constraint coincident L22.end L23.start
extrude "Extruir39" add sketch "Boceto32" along normal up to surface (6.9333 mm away) and the other way up to surface (13.8667 mm away) contours L8 L9 L34 | L16 L17 L35 | L23 L24 L37 | L32 L33 L36 bodies 2 3 4
fillet "Empalme2" radius 3 4 edges at (75, 186.5, 5) (88.0667, 186.5, 5) (-88.0667, 186.5, 5) (-75, 186.5, 5) on bodies 3
fillet "Empalme3" radius 1 8 edges at (-75, -11.5, -1.9333) (-75, -11.5, 11.9333) (75, -11.5, -1.9333) (75, -11.5, 11.9333) (75, 211.5, -1.9333) (75, 211.5, 11.9333) (-75, 211.5, -1.9333) (-75, 211.5, 11.9333) on bodies 2 3
sketch "Boceto33" plane through (0, -35.5, 0) normal (0, -1, 0) x (1, 0, 0)
  line L0 (-75, -5.4) -> (75, -5.4)
  line L1 (75, -5.4) -> (75, 15.4)
  line L2 (75, 15.4) -> (-75, 15.4)
  line L3 (-75, 15.4) -> (-75, -5.4)
  line L4 (75, -5.4) -> (75, -35.4)
  line L5 (75, -35.4) -> (50, -35.4)
  line L6 (50, -35.4) -> (35, -5.4)
  line L7 (75, 15.4) -> (75, 45.4)
  line L8 (75, 45.4) -> (50, 45.4)
  line L9 (50, 45.4) -> (35, 15.4)
  line L10 (-75, -5.4) -> (-75, -35.4)
  line L11 (-75, -35.4) -> (-50, -35.4)
  line L12 (-50, -35.4) -> (-35, -5.4)
  line L13 (-75, 15.4) -> (-75, 45.4)
  line L14 (-75, 45.4) -> (-50, 45.4)
  line L15 (-50, 45.4) -> (-35, 15.4)
  dimension "d181" = 30
  dimension "d182" = 25
  dimension "d183" = 40
  constraint coincident L0.end L1.start
  constraint perpendicular L0 L4
  constraint perpendicular L1 L5
  constraint coincident L0 L6.end
  constraint coincident L1.end L2.start
  constraint perpendicular L2 L7
  constraint perpendicular L7 L8
  constraint coincident L2 L9.end
  constraint coincident L0.start L3.end
  constraint perpendicular L0 L10
  constraint perpendicular L10 L11
  constraint coincident L0 L12.end
  constraint parallel L9 L12
  constraint coincident L2.end L3.start
  constraint perpendicular L2 L13
  constraint perpendicular L13 L14
  constraint coincident L2 L15.end
  constraint equal L5 L8
  constraint equal L4 L7
  constraint equal L4 L10
  constraint equal L5 L11
  constraint equal L8 L14
  constraint equal L7 L13
  constraint equal L6 L9
  constraint equal L9 L15
  measures "d181" distance of L0.end L4.end
  measures "d182" distance of L4.end L5.end
  measures "d183" distance of L0.end L6.end
extrude "Extruir40" add sketch "Boceto33" against normal blind 4 contours L0 L10 L11 L12 | L2 L13 L14 L15 | L0 L4 L5 L6 | L2 L7 L8 L9 bodies 2
sketch "Boceto34" plane through (-75, 0, 0) normal (-1, 0, 0) x (0, -1, 0)
  line L0 (13.9142, 15.4) -> (13.9142, 8.4667)
  line L1 (13.9142, 8.4667) -> (31.5, 8.4667)
  line L2 (31.5, 8.4667) -> (31.5, 1.5333)
  line L3 (31.5, 1.5333) -> (13.9142, 1.5333)
  line L4 (13.9142, 1.5333) -> (13.9142, -5.4)
  line L5 (13.9142, -5.4) -> (31.5, -5.4)
  line L6 (31.5, -5.4) -> (31.5, -35.4)
  line L7 (31.5, -35.4) -> (35.5, -35.4)
  line L8 (35.5, -35.4) -> (35.5, 45.4)
  line L9 (35.5, 45.4) -> (31.5, 45.4)
  line L10 (31.5, 45.4) -> (31.5, 15.4)
  line L11 (31.5, 15.4) -> (13.9142, 15.4)
  arc A0 (-26, 2.5) -> (-26, 7.5) centre (-26, 5) ccw
  line L12 (-26, 2.5) -> (-211.5, 2.5)
  arc A1 (-211.5, 7.5) -> (-211.5, 2.5) centre (-211.5, 5) ccw
  line L13 (-211.5, 7.5) -> (-26, 7.5)
  line L14 (35.5, 15.4) -> (-238.5, 15.4)
  line L15 (-238.5, 15.4) -> (-238.5, -5.4)
  line L16 (-238.5, -5.4) -> (35.5, -5.4)
  line L17 (35.5, -5.4) -> (35.5, 15.4)
  line L18 (-238.7, -5.6) -> (35.7, -5.6)
  line L19 (35.7, -5.6) -> (35.7, 15.6)
  line L20 (35.7, 15.6) -> (-238.7, 15.6)
  line L21 (-238.7, 15.6) -> (-238.7, -5.6)
  dimension "d186" = 0.2
extrude "Extruir41" add sketch "Boceto34" along normal up to surface (23.0667 mm away) contours L8 L9 L10 L20 | L6 L7 L8 L18 bodies 2
sketch "Boceto35" plane through (75, 0, 0) normal (1, 0, 0) x (0, 1, 0)
  line L0 (-13.9142, 8.4667) -> (-13.9142, 15.4)
  line L1 (-13.9142, 15.4) -> (-31.5, 15.4)
  line L2 (-31.5, 15.4) -> (-31.5, 45.4)
  line L3 (-31.5, 45.4) -> (-35.5, 45.4)
  line L4 (-35.5, 45.4) -> (-35.5, -35.4)
  line L5 (-35.5, -35.4) -> (-31.5, -35.4)
  line L6 (-31.5, -35.4) -> (-31.5, -5.4)
  line L7 (-31.5, -5.4) -> (-13.9142, -5.4)
  line L8 (-13.9142, -5.4) -> (-13.9142, 1.5333)
  line L9 (-13.9142, 1.5333) -> (-31.5, 1.5333)
  line L10 (-31.5, 1.5333) -> (-31.5, 8.4667)
  line L11 (-31.5, 8.4667) -> (-13.9142, 8.4667)
  arc A0 (26, 7.5) -> (26, 2.5) centre (26, 5) ccw
  line L12 (26, 7.5) -> (211.5, 7.5)
  arc A1 (211.5, 2.5) -> (211.5, 7.5) centre (211.5, 5) ccw
  line L13 (211.5, 2.5) -> (26, 2.5)
  line L14 (-35.5, -5.4) -> (238.5, -5.4)
  line L15 (238.5, -5.4) -> (238.5, 15.4)
  line L16 (238.5, 15.4) -> (-35.5, 15.4)
  line L17 (-35.5, 15.4) -> (-35.5, -5.4)
  line L18 (-35.7, -5.6) -> (238.7, -5.6)
  line L19 (238.7, -5.6) -> (238.7, 15.6)
  line L20 (238.7, 15.6) -> (-35.7, 15.6)
  line L21 (-35.7, 15.6) -> (-35.7, -5.6)
  dimension "d189" = 0.2
extrude "Extruir42" add sketch "Boceto35" along normal up to surface (23.0667 mm away) contours L2 L3 L4 L20 | L4 L5 L6 L18 bodies 2
sketch "Boceto36" plane through (0, 238.5, 0) normal (0, 1, 0) x (-1, 0, 0)
  line L0 (-98.0667, 15.4) -> (-98.0667, -5.4)
  line L1 (-98.0667, -5.4) -> (-75.15, -5.4)
  line L2 (-75.15, -5.4) -> (-75.15, 1.3833)
  line L3 (-75.15, 1.3833) -> (-88.2167, 1.3833)
  line L4 (-88.2167, 1.3833) -> (-88.2167, 8.6167)
  line L5 (-88.2167, 8.6167) -> (-75.15, 8.6167)
  line L6 (-75.15, 8.6167) -> (-75.15, 15.4)
  line L7 (-75.15, 15.4) -> (-98.0667, 15.4)
  line L8 (-75, 15.6) -> (-75, 15.4)
  line L9 (-75, 15.4) -> (-35, 15.4)
  line L10 (-35, 15.4) -> (-50, 45.4)
  line L11 (-50, 45.4) -> (-98.0667, 45.4)
  line L12 (-98.0667, 45.4) -> (-98.0667, 15.6)
  line L13 (-98.0667, 15.6) -> (-75, 15.6)
  line L14 (98.0667, 45.4) -> (50, 45.4)
  line L15 (50, 45.4) -> (35, 15.4)
  line L16 (35, 15.4) -> (75, 15.4)
  line L17 (75, 15.4) -> (75, 15.6)
  line L18 (75, 15.6) -> (98.0667, 15.6)
  line L19 (98.0667, 15.6) -> (98.0667, 45.4)
  line L20 (75, -5.6) -> (75, -5.4)
  line L21 (75, -5.4) -> (35, -5.4)
  line L22 (35, -5.4) -> (50, -35.4)
  line L23 (50, -35.4) -> (98.0667, -35.4)
  line L24 (98.0667, -35.4) -> (98.0667, -5.6)
  line L25 (98.0667, -5.6) -> (75, -5.6)
  line L26 (-98.0667, -35.4) -> (-50, -35.4)
  line L27 (-50, -35.4) -> (-35, -5.4)
  line L28 (-35, -5.4) -> (-75, -5.4)
  line L29 (-75, -5.4) -> (-75, -5.6)
  line L30 (-75, -5.6) -> (-98.0667, -5.6)
  line L31 (-98.0667, -5.6) -> (-98.0667, -35.4)
  line L32 (98.0667, -5.4) -> (98.0667, 15.4)
  line L33 (98.0667, 15.4) -> (75.15, 15.4)
  line L34 (75.15, 15.4) -> (75.15, 8.6167)
  line L35 (75.15, 8.6167) -> (88.2167, 8.6167)
  line L36 (88.2167, 8.6167) -> (88.2167, 1.3833)
  line L37 (88.2167, 1.3833) -> (75.15, 1.3833)
  line L38 (75.15, 1.3833) -> (75.15, -5.4)
  line L39 (75.15, -5.4) -> (98.0667, -5.4)
  line L40 (-65, 1.5333) -> (-75, 1.5333)
  line L41 (-75, 1.5333) -> (-75, -5.4)
  line L42 (-75, -5.4) -> (75, -5.4)
  line L43 (75, -5.4) -> (75, 1.5333)
  line L44 (75, 1.5333) -> (65, 1.5333)
  line L45 (65, 1.5333) -> (65, 8.4667)
  line L46 (65, 8.4667) -> (75, 8.4667)
  line L47 (75, 8.4667) -> (75, 15.4)
  line L48 (75, 15.4) -> (-75, 15.4)
  line L49 (-75, 15.4) -> (-75, 8.4667)
  line L50 (-75, 8.4667) -> (-65, 8.4667)
  line L51 (-65, 8.4667) -> (-65, 1.5333)
  circle A0 centre (-25, 5) radius 2.15
  circle A1 centre (25, 5) radius 2.15
  line L52 (70, 8.4667) -> (70, 15.4)
  line L53 (70, 1.5333) -> (70, -5.4)
  line L54 (-70, 8.4667) -> (-70, 15.4)
  line L55 (-70, 1.5333) -> (-70, -5.4)
  circle A2 centre (75, 15.6) radius 1
  circle A3 centre (75, -5.6) radius 1
  circle A4 centre (98.0667, 15.6) radius 1
  circle A5 centre (98.0667, -5.4) radius 1
  circle A6 centre (-75, 15.6) radius 1
  circle A7 centre (-75, -5.6) radius 1
  circle A8 centre (-98.0667, -5.6) radius 1
  circle A9 centre (-98.0667, 15.6) radius 1
  line L56 (-74.95, -5.6) -> (-74.95, 1.5833)
  line L57 (-74.95, 1.5833) -> (-88.0167, 1.5833)
  line L58 (-88.0167, 1.5833) -> (-88.0167, 8.4167)
  line L59 (-88.0167, 8.4167) -> (-74.95, 8.4167)
  line L60 (-74.95, 8.4167) -> (-74.95, 15.6)
  line L61 (-74.95, 15.6) -> (-98.2667, 15.6)
  line L62 (-98.2667, 15.6) -> (-98.2667, -5.6)
  line L63 (-98.2667, -5.6) -> (-74.95, -5.6)
  line L64 (74.95, 15.6) -> (74.95, 8.4167)
  line L65 (74.95, 8.4167) -> (88.0167, 8.4167)
  line L66 (88.0167, 8.4167) -> (88.0167, 1.5833)
  line L67 (88.0167, 1.5833) -> (74.95, 1.5833)
  line L68 (74.95, 1.5833) -> (74.95, -5.6)
  line L69 (74.95, -5.6) -> (98.2667, -5.6)
  line L70 (98.2667, -5.6) -> (98.2667, 15.6)
  line L71 (98.2667, 15.6) -> (74.95, 15.6)
  line L72 (70, 15.4) -> (70, 20.4)
  line L73 (70, 20.4) -> (103.2667, 20.4)
  line L74 (103.2667, 20.4) -> (103.2667, -10.4)
  line L75 (103.2667, -10.4) -> (70, -10.4)
  line L76 (70, -10.4) -> (70, -5.4)
  line L77 (0, 45.4) -> (0, -35.4)
  line L78 (50, 45.4) -> (0, 45.4)
  line L79 (50, -35.4) -> (0, -35.4)
  line L80 (0, 15.4) -> (0, -5.4)
  line L81 (103.2667, 20.4) -> (50, 45.4)
  line L82 (103.2667, -10.4) -> (50, -35.4)
  line L83 (0, 40.4) -> (47.5, 40.4)
  line L84 (47.5, 40.4) -> (90.1133, 20.4)
  line L85 (0, -30.4) -> (47.5, -30.4)
  line L86 (47.5, -30.4) -> (90.1133, -10.4)
  line L87 (70, 10.4667) -> (74.95, 10.4667)
  line L88 (70, -0.4667) -> (74.95, -0.4667)
  dimension "d192" = 2
  dimension "d193" = 2
  dimension "d194" = 2
  dimension "d195" = 2
  dimension "d196" = 2
  dimension "d197" = 2
  dimension "d198" = 2
  dimension "d199" = 2
  dimension "d200" = 0.2
  dimension "d201" = 0.2
  dimension "d202" = 5
  dimension "d203" = 5
  dimension "d204" = 5
  dimension "d205" = 5
  dimension "d206" = 5
  dimension "d207" = 2
  dimension "d208" = 2
  constraint midpoint L46 L52.start
  constraint coincident L16 L52.end
  constraint midpoint L44 L53.start
  constraint coincident L21 L53.end
  constraint midpoint L50 L54.start
  constraint coincident L48 L54.end
  constraint midpoint L40 L55.start
  constraint coincident L28 L55.end
  constraint perpendicular L50 L54
  constraint perpendicular L40 L55
  constraint perpendicular L46 L52
  constraint perpendicular L44 L53
  constraint coincident L17.end L18.start
  constraint coincident L20.start L25.end
  constraint coincident L18.end L19.start
  constraint coincident L32.start L39.end
  constraint coincident L8.start L13.end
  constraint coincident L29.end L30.start
  constraint coincident L30.end L31.start
  constraint coincident L12.end L13.start
  constraint perpendicular L16 L72
  constraint perpendicular L19 L73
  constraint perpendicular L73 L74
  constraint perpendicular L19 L75
  constraint perpendicular L75 L76
  constraint coincident L14.end L15.start
  constraint coincident L22.end L23.start
  constraint midpoint L48 L80.start
  constraint midpoint L42 L80.end
  constraint coincident L77 L80.start
  constraint perpendicular L77 L78
  constraint perpendicular L77 L79
  constraint vertical L77
  constraint coincident L77 L83.start
  constraint coincident L15 L83.end
  constraint perpendicular L77 L83
  constraint coincident L73 L84.end
  constraint coincident L77 L85.start
  constraint coincident L22 L85.end
  constraint perpendicular L77 L85
  constraint coincident L75 L86.end
  constraint parallel L81 L84
  constraint parallel L82 L86
  constraint coincident L52 L87.start
  constraint coincident L64 L87.end
  constraint perpendicular L47 L87
  constraint coincident L53 L88.start
  constraint coincident L68 L88.end
  constraint perpendicular L68 L88
  measures "d192" diameter of A2
  measures "d193" diameter of A3
  measures "d194" diameter of A4
  measures "d195" diameter of A5
  measures "d196" diameter of A6
  measures "d197" diameter of A7
  measures "d198" diameter of A8
  measures "d199" diameter of A9
  measures "d202" distance of L70 L74
  measures "d203" distance of L53.end L75.end
  measures "d204" distance of L52.end L72.end
  measures "d205" distance of L78 L83
  measures "d206" distance of L79 L85
  measures "d207" distance of L46 L87
  measures "d208" distance of L44 L88
extrude "Extruir43" add sketch "Boceto36" against normal blind 6 separate body contours L15 L77 L78 L83 | L22 L77 L79 L85 | L15 L19 L73 L81 L84 | L16 L18 L19 L48 A2 A4 L71 L72 L73 | L16 L48 L52 A2 L64 L87 | L21 L42 L53 A3 L68 L88 | L21 L24 L25 L42 A3 A5 L69 L75 L76 | L22 L24 L75 L82 L86 | L19 L73 L81 | L19 L24 A4 A5 L70 L73 L74 L75 | L24 L75 L82 makes body 7
sketch "Boceto37" plane through (0, 238.5, 0) normal (0, 1, 0) x (-1, 0, 0)
  line L0 (0, -30.4) -> (0, -35.4)
  line L1 (0, -35.4) -> (50, -35.4)
  line L2 (50, -35.4) -> (103.2667, -10.4)
  line L3 (103.2667, -10.4) -> (103.2667, 20.4)
  line L4 (103.2667, 20.4) -> (50, 45.4)
  line L5 (50, 45.4) -> (0, 45.4)
  line L6 (0, 45.4) -> (0, 40.4)
  line L7 (0, 40.4) -> (47.5, 40.4)
  line L8 (47.5, 40.4) -> (90.1133, 20.4)
  line L9 (90.1133, 20.4) -> (70, 20.4)
  line L10 (70, 20.4) -> (70, 10.4667)
  line L11 (70, 10.4667) -> (74.95, 10.4667)
  line L12 (74.95, 10.4667) -> (74.95, 14.6013)
  arc A0 (76, 15.6) -> (74.95, 14.6013) centre (75, 15.6) ccw
  line L13 (76, 15.6) -> (97.0667, 15.6)
  arc A1 (98.2667, 14.6202) -> (97.0667, 15.6) centre (98.0667, 15.6) ccw
  line L14 (98.2667, 14.6202) -> (98.2667, -4.4202)
  arc A2 (97.0869, -5.6) -> (98.2667, -4.4202) centre (98.0667, -5.4) ccw
  line L15 (97.0869, -5.6) -> (76, -5.6)
  arc A3 (74.95, -4.6013) -> (76, -5.6) centre (75, -5.6) ccw
  line L16 (74.95, -4.6013) -> (74.95, -0.4667)
  line L17 (74.95, -0.4667) -> (70, -0.4667)
  line L18 (70, -0.4667) -> (70, -10.4)
  line L19 (70, -10.4) -> (90.1133, -10.4)
  line L20 (90.1133, -10.4) -> (47.5, -30.4)
  line L21 (47.5, -30.4) -> (0, -30.4)
  line L22 (90.1133, 20.4) -> (90.1133, -10.4)
  constraint coincident L8.end L9.start
  constraint coincident L19.end L20.start